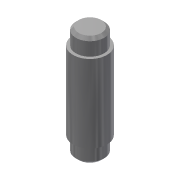
# Autodesk Inventor part: Axle
Saved by Autodesk Inventor 2022 Beta2 (Build 260130000, 130) ContinuousBuild 0
## iProperties
Created: 2007-03-01
Part Number: Axle
Document SubType Name: Modeling
Designer: MFlayler
Material: Galvanized Steel
Mass: 250.199 g
Surface Area: 63.3918 cm^2
Volume: 31.8725 cm^3
Density: 7.85 g/cm^3
Appearance: Steel
Author: MFlayler
Autodesk Inventor part; units mm, degrees
ref_plane "YZ Plane" through (0, 0, 0) normal (1, 0, 0) x (0, 1, 0)
ref_plane "XZ Plane" through (0, 0, 0) normal (0, 1, 0) x (-1, 0, 0)
ref_plane "XY Plane" through (0, 0, 0) normal (0, 0, 1) x (1, 0, 0)
sketch "Sketch1" plane through (0, 0, 0) normal (0, 0, 1) x (1, 0, 0)
  line L0 (0, 19.2) -> (0, -14.4) projected
  line L1 (-14.4, 0) -> (19.2, 0) projected
  circle A0 centre (0, 0) radius 12
  dimension "d0" = 24
  constraints: 2 point on line, 1 centre point
  measures "d0" diameter of A0
extrude "Extrusion1" add sketch "Sketch1" along normal mid plane 55
sketch "Sketch2" plane through (0, 0, 0) normal (0, 0, 1) x (1, 0, 0)
  circle A0 centre (0, 0) radius 12 projected
  circle A1 centre (0, 0) radius 12 projected
  circle A2 centre (0, 0) radius 10
  dimension "d3" = 20
  constraints: 1 centre point, 1 coincident
  measures "d3" diameter of A2
extrude "Extrusion2" add sketch "Sketch2" along normal mid plane 78 contours A2
chamfer "Chamfer1" distance 2 angle 45 2 edges at (-10, 0, 39) (-10, 0, -39)
body "Solid1"
